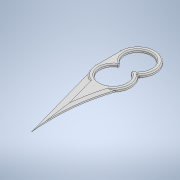
# Autodesk Inventor part: Box Cutter
Saved by Autodesk Inventor 2020 (Build 240168000, 168)
## iProperties
Created: 2020-02-13
Part Number: Box Cutter
Material: Generic
Document SubType Name: Modeling
Designer: maple
Density: 1 g/cm^3
Appearance: Default
Author: maple
Autodesk Inventor part; units mm, degrees
ref_plane "YZ Plane" through (0, 0, 0) normal (1, 0, 0) x (0, 1, 0)
ref_plane "XZ Plane" through (0, 0, 0) normal (0, 1, 0) x (-1, 0, 0)
ref_plane "XY Plane" through (0, 0, 0) normal (0, 0, 1) x (1, 0, 0)
sketch "Sketch1" plane through (0, 0, 0) normal (0, 1, 0) x (-1, 0, 0)
  circle A0 centre (0, 0) radius 9.525
  line L0 (0, 0) -> (0, -17.78)
  circle A1 centre (0, -17.78) radius 9.525
  circle A2 centre (0, 0) radius 12.7
  circle A3 centre (0, -17.78) radius 12.7
  line L1 (0, 12.7) -> (0, 63.5)
  line L2 (0, 63.5) -> (-5.08, 63.5)
  line L3 (-5.08, 63.5) -> (12.7, 0)
  arc A4 (-12.7, 0) -> (-5.08, 63.5) centre (-126.4642, 45.8589) ccw
  line L4 (12.7, 0) -> (12.7, -17.78)
  point P0 (-9.0696, -8.89)
  point P1 (10.8534, 6.595)
  point P2 (-9.7482, 8.1402)
  point P3 (-3.4196, -8.89)
  point P4 (3.4196, -8.89)
  dimension "d4" = 25.4
  dimension "d0" = 19.05
  dimension "d1" = 17.78
  dimension "d2" = 19.05
  dimension "d3" = 25.4
  dimension "d5" = 50.8
  dimension "d6" = 5.08
  constraints: 10 end point, 5 point on circle, 4 centre point, 4 coincident, 3 vertical, 1 horizontal, 3 other
  measures "d0" diameter of A0
  measures "d1" distance of L0.start L0.end
  measures "d2" diameter of A1
  measures "d3" diameter of A2
  measures "d5" distance of L1.start L1.end
  measures "d6" distance of L1.end L2.end
extrude "Extrusion1" add sketch "Sketch1" along normal blind 2.54 contours A0 A3 A2 A4 L3 | A0 A1 A2 A3 | A3 A2 A1 A0 | A2 A1 A3 | A2 L4 A3 | A2 A4 | L3 A2 | A4 L3 L1 A2 | A2 L1 L3
chamfer "Chamfer1" distance 5.08 distance2 1.27 1 edges at (-2.8867, 2.54, 35.0475) measured on face at (-2.4052, 2.54, 34.9127)
chamfer "Chamfer2" distance 5.08 distance2 1.27 1 edges at (-2.8867, 0, 35.0475) measured on face at (-2.4052, 0, 34.9127)
chamfer "Chamfer3" distance 2.54 distance2 0.762 1 edges at (5.744, 2.54, 24.1339) measured on face at (5.2519, 2.54, 24.0454)
chamfer "Chamfer4" distance 2.54 distance2 0.762 1 edges at (5.744, 0, 24.1341) measured on face at (5.2519, 0, 24.0455)
fillet "Fillet5" radius 0.762 18 edges at (-3.4196, 1.27, -8.89) (3.4196, 1.27, -8.89) (0, 2.54, 9.525) (0, 2.54, -27.305) (0, 0, -27.305) (0, 0, 9.525) (-7.9349, 0, 9.916) (-12.2296, 0, 3.4243) (4.8013, 0, -29.5374) (-12.7, 0, -8.89) (-7.9349, 2.54, 9.916) (-12.2296, 2.54, 3.4243) (4.8013, 2.54, -29.5374) (-12.7, 2.54, -8.89) (8.1042, 0, 9.7782) (12.6899, 0, -0.5056) (8.1042, 2.54, 9.7782) (12.6899, 2.54, -0.5056)
fillet "Fillet6" radius 0.762 3 edges at (9.0696, 1.27, -8.89) (8.7311, 0.2073, -8.89) (8.7311, 2.3327, -8.89)
body "Solid1"
